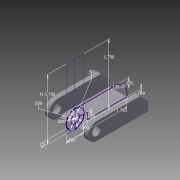
# Autodesk Inventor part: LegHolderV1
Saved by Autodesk Inventor 2014 (Build 180170000, 170)
## iProperties
Created: 2014-04-23
Part Number: LegHolderV1
Material: Generic
Document SubType Name: Modeling
Designer: Max
Density: 1 g/cm^3
Appearance: Default
Author: Max
Autodesk Inventor part; units mm, degrees
ref_plane "YZ Plane" through (0, 0, 0) normal (1, 0, 0) x (0, 1, 0)
ref_plane "XZ Plane" through (0, 0, 0) normal (0, 1, 0) x (-1, 0, 0)
ref_plane "XY Plane" through (0, 0, 0) normal (0, 0, 1) x (1, 0, 0)
sketch "Sketch1" plane through (0, 0, 0) normal (1, 0, 0) x (0, 1, 0)
  line L0 (6.35, 0) -> (44.45, 0) construction
  line L1 (44.45, 0) -> (44.45, 12.7) construction
  line L2 (44.45, 12.7) -> (0, 12.7) construction
  line L3 (0, 12.7) -> (0, 6.35)
  arc A0 (0, 6.35) -> (6.35, 0) centre (6.35, 6.35) ccw construction
  line L4 (0, 6.35) -> (44.45, 6.35) construction
  circle A1 centre (6.35, 6.35) radius 2.54 construction
  line L5 (0, 6.35) -> (3.175, 12.7) construction
  circle A2 centre (6.35, 6.35) radius 3.175
  circle A3 centre (6.35, 6.35) radius 6.35
  line L6 (0, 6.35) -> (0, -31.75)
  line L7 (12.7, 6.35) -> (12.7, -25.4)
  line L8 (1.27, -31.6863) -> (1.27, -2.54)
  line L9 (6.35, 0) -> (6.35, -2.54)
  line L10 (6.35, -2.54) -> (1.27, -2.54)
  line L11 (0, -31.75) -> (0, 6.35)
  line L12 (12.7, 6.35) -> (12.7, -19.05)
  line L13 (1.27, -31.6863) -> (1.27, -2.54)
  line L14 (1.27, -2.54) -> (6.35, -2.54)
  line L15 (6.35, -2.54) -> (6.35, 0)
  line L16 (0, -31.75) -> (6.35, -31.75)
  line L17 (6.35, -31.75) -> (12.7, -25.4)
  line L18 (6.35, -2.54) -> (6.35, 0)
  line L19 (0, 6.35) -> (12.7, 6.35)
  line L20 (12.7, 6.35) -> (12.7, -25.4)
  line L21 (6.35, -31.75) -> (12.7, -25.4)
  line L22 (6.35, -31.75) -> (0, -31.75)
  line L23 (0, -31.75) -> (0, 6.35)
  circle A4 centre (6.35, 6.35) radius 6.35
  circle A5 centre (6.35, 6.35) radius 3.175
  line L24 (6.35, 3.175) -> (6.35, -2.54)
  line L25 (6.35, -2.54) -> (1.27, -2.54)
  line L26 (1.27, -31.6863) -> (1.27, -2.54)
  line L27 (6.35, -2.54) -> (1.27, -2.54)
  line L28 (6.35, -2.54) -> (6.35, 3.175)
  circle A6 centre (6.35, 6.35) radius 6.6675
  point P0 (0, 0)
  dimension "d9" = 12.7
  dimension "d0" = 12.7
  dimension "d2" = 12.7
  dimension "d3" = 44.45
  dimension "d4" = 44.45
  dimension "d5" = 6.35
  dimension "d6" = 5.08
  dimension "d7" = 3.175
  dimension "d8" = 0.635
  dimension "d10" = 44.45
  dimension "d11" = 1.27
  dimension "d13" = 2.54
  dimension "d14" = 135
  dimension "d15" = 6.35
  dimension "d20" = 13.335
  constraints: 58 end point, 6 coincident, 5 collinear, 5 perpendicular, 5 vertical, 4 parallel, 4 point on line, 3 centre point, 2 horizontal alignment, 2 point on circle, 2 tangent, 2 vertical alignment, 1 horizontal, 1 midpoint, 8 other
  measures "d0" distance of L2.end point (0, 0)
  measures "d2" diameter of A0
  measures "d3" distance from line of L1 point (0, 0)
  measures "d4" distance from line of L1 L3.end
  measures "d5" distance of L0.start point (0, 0)
  measures "d6" diameter of A1
  measures "d7" horizontal distance of L3.end L5.end
  measures "d10" distance from line of L6.end L2
  measures "d11" distance from line of point (0, 0) L8
  measures "d13" distance from line of point (0, 0) L10
  measures "d14" angle of L7 L17
  measures "d15" horizontal distance of L16.end L7.end
  measures "d20" diameter of A6
extrude "Extrusion1" add sketch "Sketch1" along normal mid plane 31.75 contours L19 A2 L24 A3 | A3 L9 A6 L6 | A3 L19 A2 | A6 L7 L17 L16 L6 | L7 A6 L9 A3 | A3 L24 A2 L19
extrude "Extrusion2" cut sketch "Sketch1" along normal through all both and the other way through all contours L19 A2 | A2 L19
sketch "Sketch2" plane through (0, 0, 0) normal (1, 0, 0) x (0, 1, 0)
  circle A0 centre (6.35, 6.35) radius 6.6675 projected
  circle A1 centre (6.35, 6.35) radius 6.6675
  line L0 (6.35, -2.5607) -> (6.35, -0.3175)
  line L1 (12.7, 6.35) -> (12.7, -25.4) projected
  line L2 (0, -31.75) -> (0, 6.35) projected
  line L3 (6.35, -2.5607) -> (1.27, -2.5607)
  line L4 (1.27, -2.5607) -> (1.27, -31.75)
  line L5 (1.27, -31.75) -> (12.7, -31.75)
  line L6 (12.7, -31.75) -> (12.7, 4.317)
  line L7 (1.27, -2.5607) -> (1.27, 2.0315)
  point P0 (0, 0)
  dimension "d21" = 6.35
  dimension "d22" = 5.08
  constraints: 12 end point, 3 parallel, 3 point on circle, 2 perpendicular, 1 centre point, 1 coincident, 1 point on line, 1 vertical alignment, 2 other
  measures "d21" distance between parallel lines of L2 L0
  measures "d22" distance of L0.start L3.end
extrude "Extrusion3" cut sketch "Sketch2" along normal mid plane 25.4
fillet "Fillet2" radius 0.3969 2 edges at (-12.7, 3.175, 6.35) (12.7, 3.175, 6.35)
equation "\"d4\" = d3"
body "Solid1"
